Autodesk Inventor part; units mm, degrees
(part 2 of 2)
  line L348 (-0.7835, -0.4545) -> (-0.7886, -0.4573)
  line L349 (-0.7886, -0.4573) -> (-0.7936, -0.4603)
  line L350 (-0.7936, -0.4603) -> (-0.7985, -0.4636)
  line L351 (-0.7985, -0.4636) -> (-0.8034, -0.467)
  line L352 (-0.8034, -0.467) -> (-0.8083, -0.4707)
  line L353 (-0.8083, -0.4707) -> (-0.8131, -0.4745)
  line L354 (-0.8131, -0.4745) -> (-0.8178, -0.4786)
  line L355 (-0.8178, -0.4786) -> (-0.8067, -0.5276)
  line L356 (-0.8067, -0.5276) -> (-0.8006, -0.5292)
  line L357 (-0.8006, -0.5292) -> (-0.7946, -0.5306)
  line L358 (-0.7946, -0.5306) -> (-0.7887, -0.5318)
  line L359 (-0.7887, -0.5318) -> (-0.7827, -0.5328)
  line L360 (-0.7827, -0.5328) -> (-0.7769, -0.5335)
  line L361 (-0.7769, -0.5335) -> (-0.771, -0.5341)
  line L362 (-0.771, -0.5341) -> (-0.7653, -0.5344)
  line L363 (-0.7653, -0.5344) -> (-0.7596, -0.5345)
  line L364 (-0.7596, -0.5345) -> (-0.754, -0.5343)
  line L365 (-0.754, -0.5343) -> (-0.7485, -0.5338)
  line L366 (-0.7485, -0.5338) -> (-0.7432, -0.5329)
  line L367 (-0.7432, -0.5329) -> (-0.738, -0.5316)
  line L368 (-0.738, -0.5316) -> (-0.7353, -0.5311)
  line L369 (-0.7353, -0.5311) -> (-0.7326, -0.5307)
  line L370 (-0.7326, -0.5307) -> (-0.7299, -0.5305)
  line L371 (-0.7299, -0.5305) -> (-0.7284, -0.5305)
  line L372 (-0.7284, -0.5305) -> (-0.7269, -0.5307)
  line L373 (-0.7269, -0.5307) -> (-0.7254, -0.5309)
  line L374 (-0.7254, -0.5309) -> (-0.7238, -0.5313)
  line L375 (-0.7238, -0.5313) -> (-0.7221, -0.5322)
  line L376 (-0.7221, -0.5322) -> (-0.7195, -0.535)
  line L377 (-0.7195, -0.535) -> (-0.7, -0.5755)
  line L378 (-0.7, -0.5755) -> (-0.6994, -0.5792)
  line L379 (-0.6994, -0.5792) -> (-0.6999, -0.5811)
  line L380 (-0.6999, -0.5811) -> (-0.7005, -0.5826)
  line L381 (-0.7005, -0.5826) -> (-0.7013, -0.584)
  line L382 (-0.7013, -0.584) -> (-0.7021, -0.5852)
  line L383 (-0.7021, -0.5852) -> (-0.703, -0.5863)
  line L384 (-0.703, -0.5863) -> (-0.7048, -0.5884)
  line L385 (-0.7048, -0.5884) -> (-0.7068, -0.5903)
  line L386 (-0.7068, -0.5903) -> (-0.7089, -0.592)
  line L387 (-0.7089, -0.592) -> (-0.7132, -0.5952)
  line L388 (-0.7132, -0.5952) -> (-0.7172, -0.5989)
  line L389 (-0.7172, -0.5989) -> (-0.721, -0.6029)
  line L390 (-0.721, -0.6029) -> (-0.7246, -0.6071)
  line L391 (-0.7246, -0.6071) -> (-0.7281, -0.6116)
  line L392 (-0.7281, -0.6116) -> (-0.7315, -0.6163)
  line L393 (-0.7315, -0.6163) -> (-0.7347, -0.6212)
  line L394 (-0.7347, -0.6212) -> (-0.7377, -0.6263)
  line L395 (-0.7377, -0.6263) -> (-0.7406, -0.6315)
  line L396 (-0.7406, -0.6315) -> (-0.7434, -0.6369)
  line L397 (-0.7434, -0.6369) -> (-0.7461, -0.6425)
  line L398 (-0.7461, -0.6425) -> (-0.7486, -0.6482)
  line L399 (-0.7486, -0.6482) -> (-0.7172, -0.6875)
  line L400 (-0.7172, -0.6875) -> (-0.7111, -0.6863)
  line L401 (-0.7111, -0.6863) -> (-0.7051, -0.685)
  line L402 (-0.7051, -0.685) -> (-0.6992, -0.6835)
  line L403 (-0.6992, -0.6835) -> (-0.6934, -0.6818)
  line L404 (-0.6934, -0.6818) -> (-0.6878, -0.6799)
  line L405 (-0.6878, -0.6799) -> (-0.6823, -0.6779)
  line L406 (-0.6823, -0.6779) -> (-0.677, -0.6757)
  line L407 (-0.677, -0.6757) -> (-0.6719, -0.6733)
  line L408 (-0.6719, -0.6733) -> (-0.6669, -0.6707)
  line L409 (-0.6669, -0.6707) -> (-0.6622, -0.6679)
  line L410 (-0.6622, -0.6679) -> (-0.6577, -0.6648)
  line L411 (-0.6577, -0.6648) -> (-0.6536, -0.6613)
  line L412 (-0.6536, -0.6613) -> (-0.6515, -0.6597)
  line L413 (-0.6515, -0.6597) -> (-0.6492, -0.6582)
  line L414 (-0.6492, -0.6582) -> (-0.6468, -0.6568)
  line L415 (-0.6468, -0.6568) -> (-0.6455, -0.6562)
  line L416 (-0.6455, -0.6562) -> (-0.6441, -0.6557)
  line L417 (-0.6441, -0.6557) -> (-0.6426, -0.6552)
  line L418 (-0.6426, -0.6552) -> (-0.641, -0.6549)
  line L419 (-0.641, -0.6549) -> (-0.6391, -0.6549)
  line L420 (-0.6391, -0.6549) -> (-0.6355, -0.6564)
  line L421 (-0.6355, -0.6564) -> (-0.6004, -0.6844)
  line L422 (-0.6004, -0.6844) -> (-0.5982, -0.6875)
  line L423 (-0.5982, -0.6875) -> (-0.5978, -0.6894)
  line L424 (-0.5978, -0.6894) -> (-0.5977, -0.691)
  line L425 (-0.5977, -0.691) -> (-0.5978, -0.6926)
  line L426 (-0.5978, -0.6926) -> (-0.598, -0.694)
  line L427 (-0.598, -0.694) -> (-0.5983, -0.6954)
  line L428 (-0.5983, -0.6954) -> (-0.5991, -0.6981)
  line L429 (-0.5991, -0.6981) -> (-0.6001, -0.7006)
  line L430 (-0.6001, -0.7006) -> (-0.6012, -0.7031)
  line L431 (-0.6012, -0.7031) -> (-0.6037, -0.7079)
  line L432 (-0.6037, -0.7079) -> (-0.6057, -0.7129)
  line L433 (-0.6057, -0.7129) -> (-0.6074, -0.7182)
  line L434 (-0.6074, -0.7182) -> (-0.6088, -0.7236)
  line L435 (-0.6088, -0.7236) -> (-0.61, -0.7291)
  line L436 (-0.61, -0.7291) -> (-0.611, -0.7348)
  line L437 (-0.611, -0.7348) -> (-0.6118, -0.7406)
  line L438 (-0.6118, -0.7406) -> (-0.6123, -0.7465)
  line L439 (-0.6123, -0.7465) -> (-0.6127, -0.7525)
  line L440 (-0.6127, -0.7525) -> (-0.6128, -0.7586)
  line L441 (-0.6128, -0.7586) -> (-0.6128, -0.7647)
  line L442 (-0.6128, -0.7647) -> (-0.6126, -0.771)
  line L443 (-0.6126, -0.771) -> (-0.5673, -0.7928)
  line L444 (-0.5673, -0.7928) -> (-0.5623, -0.7891)
  line L445 (-0.5623, -0.7891) -> (-0.5575, -0.7852)
  line L446 (-0.5575, -0.7852) -> (-0.5528, -0.7813)
  line L447 (-0.5528, -0.7813) -> (-0.5483, -0.7773)
  line L448 (-0.5483, -0.7773) -> (-0.5441, -0.7732)
  line L449 (-0.5441, -0.7732) -> (-0.54, -0.769)
  line L450 (-0.54, -0.769) -> (-0.5362, -0.7647)
  line L451 (-0.5362, -0.7647) -> (-0.5326, -0.7603)
  line L452 (-0.5326, -0.7603) -> (-0.5292, -0.7558)
  line L453 (-0.5292, -0.7558) -> (-0.5262, -0.7512)
  line L454 (-0.5262, -0.7512) -> (-0.5235, -0.7465)
  line L455 (-0.5235, -0.7465) -> (-0.5213, -0.7416)
  line L456 (-0.5213, -0.7416) -> (-0.5201, -0.7392)
  line L457 (-0.5201, -0.7392) -> (-0.5187, -0.7368)
  line L458 (-0.5187, -0.7368) -> (-0.5171, -0.7345)
  line L459 (-0.5171, -0.7345) -> (-0.5162, -0.7334)
  line L460 (-0.5162, -0.7334) -> (-0.5152, -0.7323)
  line L461 (-0.5152, -0.7323) -> (-0.5141, -0.7313)
  line L462 (-0.5141, -0.7313) -> (-0.5127, -0.7304)
  line L463 (-0.5127, -0.7304) -> (-0.511, -0.7295)
  line L464 (-0.511, -0.7295) -> (-0.5072, -0.7293)
  line L465 (-0.5072, -0.7293) -> (-0.4634, -0.7393)
  line L466 (-0.4634, -0.7393) -> (-0.4601, -0.7411)
  line L467 (-0.4601, -0.7411) -> (-0.4589, -0.7426)
  line L468 (-0.4589, -0.7426) -> (-0.4581, -0.7441)
  line L469 (-0.4581, -0.7441) -> (-0.4575, -0.7455)
  line L470 (-0.4575, -0.7455) -> (-0.4571, -0.7469)
  line L471 (-0.4571, -0.7469) -> (-0.4567, -0.7483)
  line L472 (-0.4567, -0.7483) -> (-0.4563, -0.7511)
  line L473 (-0.4563, -0.7511) -> (-0.4561, -0.7538)
  line L474 (-0.4561, -0.7538) -> (-0.456, -0.7565)
  line L475 (-0.456, -0.7565) -> (-0.4561, -0.7618)
  line L476 (-0.4561, -0.7618) -> (-0.4558, -0.7673)
  line L477 (-0.4558, -0.7673) -> (-0.455, -0.7727)
  line L478 (-0.455, -0.7727) -> (-0.454, -0.7782)
  line L479 (-0.454, -0.7782) -> (-0.4526, -0.7837)
  line L480 (-0.4526, -0.7837) -> (-0.4511, -0.7893)
  line L481 (-0.4511, -0.7893) -> (-0.4492, -0.7948)
  line L482 (-0.4492, -0.7948) -> (-0.4472, -0.8004)
  line L483 (-0.4472, -0.8004) -> (-0.4449, -0.8059)
  line L484 (-0.4449, -0.8059) -> (-0.4424, -0.8115)
  line L485 (-0.4424, -0.8115) -> (-0.4397, -0.817)
  line L486 (-0.4397, -0.817) -> (-0.4368, -0.8226)
  line L487 (-0.4368, -0.8226) -> (-0.3865, -0.8226)
  line L488 (-0.3865, -0.8226) -> (-0.3836, -0.817)
  line L489 (-0.3836, -0.817) -> (-0.3809, -0.8115)
  line L490 (-0.3809, -0.8115) -> (-0.3784, -0.8059)
  line L491 (-0.3784, -0.8059) -> (-0.3762, -0.8004)
  line L492 (-0.3762, -0.8004) -> (-0.3741, -0.7948)
  line L493 (-0.3741, -0.7948) -> (-0.3723, -0.7893)
  line L494 (-0.3723, -0.7893) -> (-0.3707, -0.7837)
  line L495 (-0.3707, -0.7837) -> (-0.3694, -0.7782)
  line L496 (-0.3694, -0.7782) -> (-0.3683, -0.7727)
  line L497 (-0.3683, -0.7727) -> (-0.3676, -0.7673)
  line L498 (-0.3676, -0.7673) -> (-0.3672, -0.7618)
  line L499 (-0.3672, -0.7618) -> (-0.3673, -0.7565)
  line L500 (-0.3673, -0.7565) -> (-0.3673, -0.7538)
  line L501 (-0.3673, -0.7538) -> (-0.367, -0.7511)
  line L502 (-0.367, -0.7511) -> (-0.3666, -0.7483)
  line L503 (-0.3666, -0.7483) -> (-0.3663, -0.7469)
  line L504 (-0.3663, -0.7469) -> (-0.3658, -0.7455)
  line L505 (-0.3658, -0.7455) -> (-0.3652, -0.7441)
  line L506 (-0.3652, -0.7441) -> (-0.3644, -0.7426)
  line L507 (-0.3644, -0.7426) -> (-0.3633, -0.7411)
  line L508 (-0.3633, -0.7411) -> (-0.3599, -0.7393)
  line L509 (-0.3599, -0.7393) -> (-0.3161, -0.7293)
  line L510 (-0.3161, -0.7293) -> (-0.3123, -0.7295)
  line L511 (-0.3123, -0.7295) -> (-0.3106, -0.7304)
  line L512 (-0.3106, -0.7304) -> (-0.3093, -0.7313)
  line L513 (-0.3093, -0.7313) -> (-0.3081, -0.7323)
  line L514 (-0.3081, -0.7323) -> (-0.3071, -0.7334)
  line L515 (-0.3071, -0.7334) -> (-0.3062, -0.7345)
  line L516 (-0.3062, -0.7345) -> (-0.3046, -0.7368)
  line L517 (-0.3046, -0.7368) -> (-0.3032, -0.7392)
  line L518 (-0.3032, -0.7392) -> (-0.302, -0.7416)
  line L519 (-0.302, -0.7416) -> (-0.2998, -0.7465)
  line L520 (-0.2998, -0.7465) -> (-0.2971, -0.7512)
  line L521 (-0.2971, -0.7512) -> (-0.2941, -0.7558)
  line L522 (-0.2941, -0.7558) -> (-0.2908, -0.7603)
  line L523 (-0.2908, -0.7603) -> (-0.2872, -0.7647)
  line L524 (-0.2872, -0.7647) -> (-0.2833, -0.769)
  line L525 (-0.2833, -0.769) -> (-0.2793, -0.7732)
  line L526 (-0.2793, -0.7732) -> (-0.275, -0.7773)
  line L527 (-0.275, -0.7773) -> (-0.2705, -0.7813)
  line L528 (-0.2705, -0.7813) -> (-0.2659, -0.7852)
  line L529 (-0.2659, -0.7852) -> (-0.261, -0.7891)
  line L530 (-0.261, -0.7891) -> (-0.256, -0.7928)
  line L531 (-0.256, -0.7928) -> (-0.2107, -0.771)
  line L532 (-0.2107, -0.771) -> (-0.2105, -0.7647)
  line L533 (-0.2105, -0.7647) -> (-0.2105, -0.7586)
  line L534 (-0.2105, -0.7586) -> (-0.2107, -0.7525)
  line L535 (-0.2107, -0.7525) -> (-0.211, -0.7465)
  line L536 (-0.211, -0.7465) -> (-0.2116, -0.7406)
  line L537 (-0.2116, -0.7406) -> (-0.2123, -0.7348)
  line L538 (-0.2123, -0.7348) -> (-0.2133, -0.7291)
  line L539 (-0.2133, -0.7291) -> (-0.2145, -0.7236)
  line L540 (-0.2145, -0.7236) -> (-0.2159, -0.7182)
  line L541 (-0.2159, -0.7182) -> (-0.2176, -0.7129)
  line L542 (-0.2176, -0.7129) -> (-0.2197, -0.7079)
  line L543 (-0.2197, -0.7079) -> (-0.2221, -0.7031)
  line L544 (-0.2221, -0.7031) -> (-0.2232, -0.7006)
  line L545 (-0.2232, -0.7006) -> (-0.2242, -0.6981)
  line L546 (-0.2242, -0.6981) -> (-0.225, -0.6954)
  line L547 (-0.225, -0.6954) -> (-0.2253, -0.694)
  line L548 (-0.2253, -0.694) -> (-0.2255, -0.6926)
  line L549 (-0.2255, -0.6926) -> (-0.2256, -0.691)
  line L550 (-0.2256, -0.691) -> (-0.2255, -0.6894)
  line L551 (-0.2255, -0.6894) -> (-0.2251, -0.6875)
  line L552 (-0.2251, -0.6875) -> (-0.2229, -0.6844)
  line L553 (-0.2229, -0.6844) -> (-0.1878, -0.6564)
  line L554 (-0.1878, -0.6564) -> (-0.1843, -0.6549)
  line L555 (-0.1843, -0.6549) -> (-0.1823, -0.6549)
  line L556 (-0.1823, -0.6549) -> (-0.1807, -0.6552)
  line L557 (-0.1807, -0.6552) -> (-0.1792, -0.6557)
  line L558 (-0.1792, -0.6557) -> (-0.1779, -0.6562)
  line L559 (-0.1779, -0.6562) -> (-0.1766, -0.6568)
  line L560 (-0.1766, -0.6568) -> (-0.1741, -0.6582)
  line L561 (-0.1741, -0.6582) -> (-0.1719, -0.6597)
  line L562 (-0.1719, -0.6597) -> (-0.1697, -0.6613)
  line L563 (-0.1697, -0.6613) -> (-0.1656, -0.6648)
  line L564 (-0.1656, -0.6648) -> (-0.1612, -0.6679)
  line L565 (-0.1612, -0.6679) -> (-0.1564, -0.6707)
  line L566 (-0.1564, -0.6707) -> (-0.1515, -0.6733)
  line L567 (-0.1515, -0.6733) -> (-0.1463, -0.6757)
  line L568 (-0.1463, -0.6757) -> (-0.141, -0.6779)
  line L569 (-0.141, -0.6779) -> (-0.1355, -0.6799)
  line L570 (-0.1355, -0.6799) -> (-0.1299, -0.6818)
  line L571 (-0.1299, -0.6818) -> (-0.1241, -0.6835)
  line L572 (-0.1241, -0.6835) -> (-0.1182, -0.685)
  line L573 (-0.1182, -0.685) -> (-0.1122, -0.6863)
  line L574 (-0.1122, -0.6863) -> (-0.1061, -0.6875)
  line L575 (-0.1061, -0.6875) -> (-0.0747, -0.6482)
  line L576 (-0.0747, -0.6482) -> (-0.0773, -0.6425)
  line L577 (-0.0773, -0.6425) -> (-0.0799, -0.6369)
  line L578 (-0.0799, -0.6369) -> (-0.0827, -0.6315)
  line L579 (-0.0827, -0.6315) -> (-0.0856, -0.6263)
  line L580 (-0.0856, -0.6263) -> (-0.0887, -0.6212)
  line L581 (-0.0887, -0.6212) -> (-0.0919, -0.6163)
  line L582 (-0.0919, -0.6163) -> (-0.0952, -0.6116)
  line L583 (-0.0952, -0.6116) -> (-0.0987, -0.6071)
  line L584 (-0.0987, -0.6071) -> (-0.1023, -0.6029)
  line L585 (-0.1023, -0.6029) -> (-0.1061, -0.5989)
  line L586 (-0.1061, -0.5989) -> (-0.1102, -0.5952)
  line L587 (-0.1102, -0.5952) -> (-0.1144, -0.592)
  line L588 (-0.1144, -0.592) -> (-0.1165, -0.5903)
  line L589 (-0.1165, -0.5903) -> (-0.1185, -0.5884)
  line L590 (-0.1185, -0.5884) -> (-0.1204, -0.5863)
  line L591 (-0.1204, -0.5863) -> (-0.1212, -0.5852)
  line L592 (-0.1212, -0.5852) -> (-0.1221, -0.584)
  line L593 (-0.1221, -0.584) -> (-0.1228, -0.5826)
  line L594 (-0.1228, -0.5826) -> (-0.1235, -0.5811)
  line L595 (-0.1235, -0.5811) -> (-0.1239, -0.5792)
  line L596 (-0.1239, -0.5792) -> (-0.1233, -0.5755)
  line L597 (-0.1233, -0.5755) -> (-0.1038, -0.535)
  line L598 (-0.1038, -0.535) -> (-0.1012, -0.5322)
  line L599 (-0.1012, -0.5322) -> (-0.0995, -0.5313)
  line L600 (-0.0995, -0.5313) -> (-0.0979, -0.5309)
  line L601 (-0.0979, -0.5309) -> (-0.0964, -0.5307)
  line L602 (-0.0964, -0.5307) -> (-0.0949, -0.5305)
  line L603 (-0.0949, -0.5305) -> (-0.0935, -0.5305)
  line L604 (-0.0935, -0.5305) -> (-0.0907, -0.5307)
  line L605 (-0.0907, -0.5307) -> (-0.088, -0.5311)
  line L606 (-0.088, -0.5311) -> (-0.0854, -0.5316)
  line L607 (-0.0854, -0.5316) -> (-0.0802, -0.5329)
  line L608 (-0.0802, -0.5329) -> (-0.0748, -0.5338)
  line L609 (-0.0748, -0.5338) -> (-0.0693, -0.5343)
  line L610 (-0.0693, -0.5343) -> (-0.0637, -0.5345)
  line L611 (-0.0637, -0.5345) -> (-0.058, -0.5344)
  line L612 (-0.058, -0.5344) -> (-0.0523, -0.5341)
  line L613 (-0.0523, -0.5341) -> (-0.0465, -0.5335)
  line L614 (-0.0465, -0.5335) -> (-0.0406, -0.5328)
  line L615 (-0.0406, -0.5328) -> (-0.0347, -0.5318)
  line L616 (-0.0347, -0.5318) -> (-0.0287, -0.5306)
  line L617 (-0.0287, -0.5306) -> (-0.0227, -0.5292)
  line L618 (-0.0227, -0.5292) -> (-0.0167, -0.5276)
  line L619 (-0.0167, -0.5276) -> (-0.0055, -0.4786)
  line L620 (-0.0055, -0.4786) -> (-0.0102, -0.4745)
  line L621 (-0.0102, -0.4745) -> (-0.015, -0.4707)
  line L622 (-0.015, -0.4707) -> (-0.0199, -0.467)
  line L623 (-0.0199, -0.467) -> (-0.0248, -0.4636)
  line L624 (-0.0248, -0.4636) -> (-0.0298, -0.4603)
  line L625 (-0.0298, -0.4603) -> (-0.0348, -0.4573)
  line L626 (-0.0348, -0.4573) -> (-0.0398, -0.4545)
  line L627 (-0.0398, -0.4545) -> (-0.0449, -0.452)
  line L628 (-0.0449, -0.452) -> (-0.05, -0.4497)
  line L629 (-0.05, -0.4497) -> (-0.0552, -0.4478)
  line L630 (-0.0552, -0.4478) -> (-0.0604, -0.4462)
  line L631 (-0.0604, -0.4462) -> (-0.0656, -0.4451)
  line L632 (-0.0656, -0.4451) -> (-0.0682, -0.4445)
  line L633 (-0.0682, -0.4445) -> (-0.0708, -0.4437)
  line L634 (-0.0708, -0.4437) -> (-0.0734, -0.4426)
  line L635 (-0.0734, -0.4426) -> (-0.0747, -0.442)
  line L636 (-0.0747, -0.442) -> (-0.076, -0.4413)
  line L637 (-0.076, -0.4413) -> (-0.0772, -0.4404)
  line L638 (-0.0772, -0.4404) -> (-0.0785, -0.4393)
  line L639 (-0.0785, -0.4393) -> (-0.0797, -0.4378)
  circle A0 centre (-0.4114, -0.4118) radius 0.1
  point P0 (0, 0)
  dimension "d2" = 0.2
  constraints: 1 centre point
  measures "d2" diameter of A0
extrude "Extrusion2" cut sketch "Sketch2" against normal blind 1 contours A0
body "Solid1"
